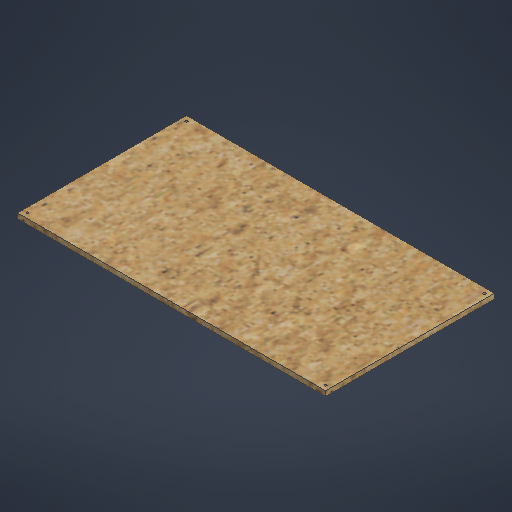
# Autodesk Inventor part: CaraSuperior
Saved by Autodesk Inventor 2026.2 (Build 302298010, 298A)
## iProperties
Created: 2026-04-15
Part Number: CaraSuperior
Material: Generic
Document SubType Name: Modeling
Designer: grego
Density: 1 g/cm^3
Appearance: Default
Author: grego
Autodesk Inventor part; units mm, degrees
ref_plane "YZ Plane" through (0, 0, 0) normal (1, 0, 0) x (0, 1, 0)
ref_plane "XZ Plane" through (0, 0, 0) normal (0, 1, 0) x (-1, 0, 0)
ref_plane "XY Plane" through (0, 0, 0) normal (0, 0, 1) x (1, 0, 0)
sketch "Sketch1" plane through (0, 0, 0) normal (0, 1, 0) x (-1, 0, 0)
  line L0 (-310, 150) -> (310, 150)
  line L1 (310, 150) -> (310, -190)
  line L2 (310, -190) -> (-310, -190)
  line L3 (-310, -190) -> (-310, 150)
  line L4 (-300, -180) -> (300, -180)
  line L5 (300, -180) -> (300, 140)
  line L6 (300, 140) -> (-300, 140)
  line L7 (-300, 140) -> (-300, -180)
  circle A0 centre (300, -180) radius 2.5
  circle A1 centre (-300, -180) radius 2.5
  circle A2 centre (-300, 140) radius 2.5
  circle A3 centre (300, 140) radius 2.5
  point P0 (0, 0)
  dimension "d0" = 620
  dimension "d1" = 340
  dimension "d2" = 10
  dimension "d3" = 5
  dimension "d4" = 5
  dimension "d5" = 5
  dimension "d6" = 5
  constraints: 16 end point, 4 centre point, 4 coincident, 4 parallel, 2 perpendicular, 1 horizontal, 3 other
  measures "d0" distance of L1.end L2.end
  measures "d1" distance of L0.end L1.end
  measures "d2" distance between parallel lines of L2 L4
  measures "d3" diameter of A0
  measures "d4" diameter of A1
  measures "d5" diameter of A2
  measures "d6" diameter of A3
extrude "Extrusion1" add sketch "Sketch1" along normal blind 10 contours L0 L1 L2 L3 | A1 L7 A2 L6 A3 L5 A0 L4
body "Solid1"
